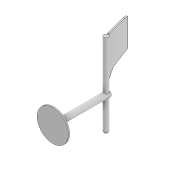
# Autodesk Inventor part: direzione del vento
Saved by Autodesk Inventor 2022 (Build 260153000, 153)
## iProperties
Created: 2025-08-06
Part Number: direzione del vento
Material: Generic
Document SubType Name: Modeling
Designer: sacchie
Density: 1 g/cm^3
Appearance: Default
Author: sacchie
Autodesk Inventor part; units mm, degrees
ref_plane "YZ Plane" through (0, 0, 0) normal (1, 0, 0) x (0, 1, 0)
ref_plane "XZ Plane" through (0, 0, 0) normal (0, 1, 0) x (-1, 0, 0)
ref_plane "XY Plane" through (0, 0, 0) normal (0, 0, 1) x (1, 0, 0)
sketch "Sketch1" plane through (0, 0, 0) normal (0, 0, 1) x (1, 0, 0)
  circle A0 centre (0, 0) radius 40
  dimension "d0" = 80
  constraints: 1 centre point, 1 coincident
  measures "d0" diameter of A0
extrude "Extrusion1" add sketch "Sketch1" along normal blind 3
sketch "Sketch2" plane through (0, 0, 3) normal (0, 0, 1) x (1, 0, 0)
  circle A0 centre (0, 0) radius 7.5
  dimension "d3" = 15
  constraints: 1 centre point, 1 coincident
  measures "d3" diameter of A0
extrude "Extrusion2" add sketch "Sketch2" against normal blind 142
sketch "Sketch3" plane through (0, 0, 0) normal (0, 1, 0) x (-1, 0, 0)
  circle A0 centre (0, -133) radius 6
  line L0 (-7.5, -139) -> (7.5, -139) projected
  line L1 (7.5, -139) -> (-7.5, -139)
  point P0 (0, 0)
  dimension "d6" = 12
  constraints: 2 end point, 1 centre point, 1 collinear, 1 tangent
  measures "d6" diameter of A0
extrude "Extrusion3" add sketch "Sketch3" along normal blind 130 and the other way blind 85
fillet "Fillet1" radius 6 1 edges at (6, -85, -133)
sketch "Sketch4" plane through (0, 0, 0) normal (1, 0, 0) x (0, 1, 0)
  line L0 (-7.5, -139) -> (7.5, -139) projected
  line L1 (0, -139) -> (147, -139)
  line L2 (147, -139) -> (147, -187)
  line L3 (147, -187) -> (0, -187)
  line L4 (0, -187) -> (0, -139)
  line L5 (147, -178.2918) -> (122.4089, -110.7284)
  line L6 (147, -178.2918) -> (218.8994, -178.2918) construction
  line L7 (7.5, -139) -> (130, -139) projected
  line L8 (32.4283, -139) -> (53.9618, -149.3242)
  line L9 (53.9618, -149.3242) -> (77.25, -187)
  line L10 (131.293, -135.1372) -> (26.6385, -135.1372)
  line L11 (32.4283, -139) -> (23.511, -135.1372)
  line L12 (23.511, -135.1372) -> (26.6385, -135.1372)
  point P0 (0, 0)
  point P1 (132.699, -139)
  dimension "d12" = 147
  dimension "d13" = 48
  dimension "d14" = 110
  constraints: 22 end point, 4 horizontal, 4 point on line, 2 parallel, 1 equal length, 1 midpoint, 1 perpendicular
  measures "d12" distance of L2.end L3.end
  measures "d13" distance of L1.end L2.end
  measures "d14" angle of L6 L5
extrude "Extrusion4" add sketch "Sketch4" along normal mid plane 4 contours L1 L5 L2 L3 L9 L8
body "Solid1"
